Autodesk Fusion 360 part; units mm, degrees
(part 6 of 25)
  arc A2244 (43.1915, 31.5347) -> (43.1519, 31.5843) centre (43.1717, 31.5595) ccw
  arc A2245 (10.8585, 39.8209) -> (11.1125, 39.4716) centre (11.2256, 39.8209) ccw
  arc A2246 (43.2035, 31.5595) -> (43.14, 31.5595) centre (43.1717, 31.5595) ccw
  line L711 (42.8542, 31.3055) -> (43.1717, 31.5595)
  arc A2247 (42.037, 30.8928) -> (42.037, 30.9563) centre (42.037, 30.9246) ccw
  arc A2248 (42.037, 30.9563) -> (42.037, 30.8928) centre (42.037, 30.9246) ccw
  arc A2249 (23.3362, 25.2095) -> (23.2728, 25.2095) centre (23.3045, 25.2095) ccw
  arc A2250 (41.7195, 31.5912) -> (41.7195, 31.5278) centre (41.7195, 31.5595) ccw
  arc A2251 (42.8542, 30.4483) -> (42.8542, 30.3848) centre (42.8542, 30.4166) ccw
  arc A2252 (23.8454, 26.1303) -> (23.8454, 26.0668) centre (23.8454, 26.0985) ccw
  arc A2253 (24.2264, 26.1303) -> (24.2264, 26.0668) centre (24.2264, 26.0985) ccw
  arc A2254 (23.3362, 26.0985) -> (23.2728, 26.0985) centre (23.3045, 26.0985) ccw
  arc A2255 (42.037, 30.9245) -> (42.037, 31.5595) centre (42.037, 31.242) ccw
  arc A2256 (42.037, 31.5912) -> (42.037, 31.5278) centre (42.037, 31.5595) ccw
  line L712 (43.9972, 31.3055) -> (44.3147, 31.5595)
  line L713 (23.8454, 24.9555) -> (24.1629, 24.9555)
  arc A2257 (24.1629, 24.9238) -> (24.1629, 24.9872) centre (24.1629, 24.9555) ccw
  line L714 (23.3045, 26.0985) -> (23.3045, 25.2095)
  line L715 (43.1717, 31.5595) -> (43.1717, 30.4165)
  line L716 (42.8542, 30.4165) -> (43.4892, 30.4165)
  arc A2258 (42.8344, 31.3303) -> (42.874, 31.2807) centre (42.8542, 31.3055) ccw
  arc A2259 (42.3261, 30.4023) -> (42.3829, 30.4307) centre (42.3545, 30.4165) ccw
  arc A2260 (42.1289, 30.9387) -> (42.0721, 30.9103) centre (42.1005, 30.9245) ccw
  arc A2261 (23.0505, 24.9872) -> (23.0505, 24.9238) centre (23.0505, 24.9555) ccw
  arc A2262 (44.3465, 31.5595) -> (44.283, 31.5595) centre (44.3147, 31.5595) ccw
  arc A2263 (24.1629, 24.9555) -> (24.1629, 25.5905) centre (24.1629, 25.273) ccw
  arc A2264 (44.3345, 31.5347) -> (44.2949, 31.5843) centre (44.3147, 31.5595) ccw
  arc A2265 (41.6878, 30.4165) -> (41.7513, 30.4165) centre (41.7196, 30.4165) ccw
  arc A2266 (24.2264, 25.6223) -> (24.2264, 25.5588) centre (24.2264, 25.5906) ccw
  arc A2267 (24.2264, 25.5905) -> (24.2264, 26.0985) centre (24.2264, 25.8445) ccw
  line L717 (41.7195, 31.5595) -> (42.037, 31.5595)
  arc A2268 (11.9809, 39.4474) -> (12.0221, 39.4958) centre (12.0015, 39.4716) ccw
  arc A2269 (43.14, 30.4165) -> (43.2035, 30.4165) centre (43.1717, 30.4165) ccw
  arc A2270 (71.2481, 44.0055) -> (71.3116, 44.0055) centre (71.2798, 44.0055) ccw
  arc A2271 (23.8454, 24.9872) -> (23.8454, 24.9238) centre (23.8454, 24.9555) ccw
  arc A2272 (71.4704, 44.2278) -> (71.4704, 44.2913) centre (71.4704, 44.2596) ccw
  arc A2273 (44.283, 30.4165) -> (44.3465, 30.4165) centre (44.3147, 30.4165) ccw
  line L718 (24.2264, 25.5905) -> (23.9724, 25.5905)
  arc A2274 (23.2728, 25.2095) -> (23.3362, 25.2095) centre (23.3045, 25.2095) ccw
  arc A2275 (70.0405, 44.0373) -> (70.0405, 43.9738) centre (70.0405, 44.0055) ccw
  arc A2276 (56.1034, 43.8468) -> (56.1034, 43.9103) centre (56.1034, 43.8786) ccw
  arc A2277 (55.5636, 43.053) -> (55.6271, 43.053) centre (55.5954, 43.053) ccw
  arc A2278 (56.2621, 43.1165) -> (56.1986, 43.1165) centre (56.2304, 43.1165) ccw
  arc A2279 (56.2304, 43.1165) -> (55.9764, 43.3705) centre (55.9764, 43.1165) ccw
  arc A2280 (55.6271, 43.053) -> (55.5636, 43.053) centre (55.5954, 43.053) ccw
  arc A2281 (70.0405, 43.9738) -> (70.0405, 44.0373) centre (70.0405, 44.0055) ccw
  line L719 (55.0545, 43.8785) -> (55.0545, 42.9895)
  arc A2282 (71.2164, 31.3055) -> (71.4704, 31.5595) centre (71.2164, 31.5595) ccw
  arc A2283 (55.9764, 43.3387) -> (55.9764, 43.4023) centre (55.9764, 43.3705) ccw
  arc A2284 (70.0405, 44.0055) -> (70.2945, 44.2595) centre (70.0405, 44.2595) ccw
  arc A2285 (70.8048, 44.2682) -> (70.8659, 44.2508) centre (70.8354, 44.2595) ccw
  line L720 (70.8354, 31.9405) -> (70.8354, 32.4485)
  line L721 (70.8354, 44.2595) -> (71.4704, 44.2595)
  arc A2286 (70.3263, 32.4485) -> (70.2627, 32.4485) centre (70.2945, 32.4485) ccw
  line L722 (70.8354, 31.3055) -> (71.2164, 31.3055)
  line L723 (70.8354, 32.4485) -> (71.4704, 32.4485)
  arc A2287 (71.2164, 31.9088) -> (71.2164, 31.9722) centre (71.2164, 31.9405) ccw
  arc A2288 (70.3263, 31.5595) -> (70.2627, 31.5595) centre (70.2945, 31.5595) ccw
  arc A2289 (71.4704, 31.6865) -> (71.2164, 31.9405) centre (71.2164, 31.6865) ccw
  arc A2290 (71.4704, 32.4168) -> (71.4704, 32.4803) centre (71.4704, 32.4486) ccw
  line L724 (70.0405, 31.3055) -> (69.9135, 31.3055)
  arc A2291 (70.8036, 31.9405) -> (70.8671, 31.9405) centre (70.8354, 31.9405) ccw
  arc A2292 (70.8354, 44.2913) -> (70.8354, 44.2278) centre (70.8354, 44.2596) ccw
  arc A2293 (70.0405, 31.2738) -> (70.0405, 31.3373) centre (70.0405, 31.3056) ccw
  arc A2294 (71.4386, 31.6865) -> (71.5021, 31.6865) centre (71.4703, 31.6865) ccw
  arc A2295 (55.5954, 43.053) -> (56.2304, 43.053) centre (55.9129, 43.053) ccw
  line L725 (30.2566, 39.8145) -> (30.2566, 38.9255)
  line L726 (55.5954, 43.053) -> (55.5954, 43.3705)
  arc A2296 (56.1986, 43.053) -> (56.2621, 43.053) centre (56.2304, 43.053) ccw
  arc A2297 (55.0228, 42.9895) -> (55.0863, 42.9895) centre (55.0546, 42.9895) ccw
  arc A2298 (56.2621, 43.053) -> (56.1986, 43.053) centre (56.2304, 43.053) ccw
  arc A2299 (55.5954, 43.4023) -> (55.5954, 43.3387) centre (55.5954, 43.3705) ccw
  arc A2300 (71.3116, 44.5135) -> (71.2481, 44.5135) centre (71.2798, 44.5135) ccw
  arc A2301 (55.5636, 43.3705) -> (55.6271, 43.3705) centre (55.5954, 43.3705) ccw
  arc A2302 (54.8005, 42.7673) -> (54.8005, 42.7037) centre (54.8005, 42.7355) ccw
  arc A2303 (70.2627, 44.2595) -> (70.3263, 44.2595) centre (70.2945, 44.2595) ccw
  arc A2304 (71.2164, 31.2738) -> (71.2164, 31.3373) centre (71.2164, 31.3056) ccw
  arc A2305 (70.8671, 32.4485) -> (70.8036, 32.4485) centre (70.8354, 32.4485) ccw
  arc A2306 (71.4386, 31.5595) -> (71.5021, 31.5595) centre (71.4703, 31.5595) ccw
  arc A2307 (70.0405, 31.3373) -> (70.0405, 31.2738) centre (70.0405, 31.3056) ccw
  arc A2308 (71.2164, 31.3373) -> (71.2164, 31.2738) centre (71.2164, 31.3056) ccw
  arc A2309 (70.8354, 32.4803) -> (70.8354, 32.4168) centre (70.8354, 32.4486) ccw
  arc A2310 (55.0863, 42.9895) -> (55.0228, 42.9895) centre (55.0546, 42.9895) ccw
  arc A2311 (69.9135, 44.0373) -> (69.9135, 43.9738) centre (69.9135, 44.0055) ccw
  line L727 (55.5954, 43.3705) -> (55.9764, 43.3705)
  arc A2312 (71.5021, 31.5595) -> (71.4386, 31.5595) centre (71.4703, 31.5595) ccw
  arc A2313 (55.6271, 43.3705) -> (55.5636, 43.3705) centre (55.5954, 43.3705) ccw
  arc A2314 (71.2164, 31.9722) -> (71.2164, 31.9088) centre (71.2164, 31.9405) ccw
  arc A2315 (69.9135, 31.3373) -> (69.9135, 31.2738) centre (69.9135, 31.3056) ccw
  line L728 (70.0405, 44.0055) -> (69.9135, 44.0055)
  line L729 (71.2164, 31.9405) -> (70.8354, 31.9405)
  arc A2316 (70.8354, 31.3373) -> (70.8354, 31.2738) centre (70.8354, 31.3056) ccw
  arc A2317 (54.8005, 42.7037) -> (54.8005, 42.7673) centre (54.8005, 42.7355) ccw
  arc A2318 (71.5021, 31.6865) -> (71.4386, 31.6865) centre (71.4703, 31.6865) ccw
  arc A2319 (56.1986, 43.1165) -> (56.2621, 43.1165) centre (56.2304, 43.1165) ccw
  arc A2320 (70.2627, 31.5595) -> (70.3263, 31.5595) centre (70.2945, 31.5595) ccw
  arc A2321 (55.0863, 43.8785) -> (55.0228, 43.8785) centre (55.0546, 43.8785) ccw
  arc A2322 (54.8005, 42.7355) -> (55.0545, 42.9895) centre (54.8005, 42.9895) ccw
  line L730 (71.4704, 31.5595) -> (71.4704, 31.6865)
  arc A2323 (70.8354, 31.9722) -> (70.8354, 31.9088) centre (70.8354, 31.9405) ccw
  arc A2324 (70.0405, 31.3055) -> (70.2945, 31.5595) centre (70.0405, 31.5595) ccw
  arc A2325 (55.9764, 43.4023) -> (55.9764, 43.3387) centre (55.9764, 43.3705) ccw
  arc A2326 (58.1354, 31.623) -> (58.7704, 31.623) centre (58.4529, 31.623) ccw
  line L731 (30.7975, 39.8145) -> (31.4325, 39.8145)
  arc A2327 (54.6735, 42.7673) -> (54.6735, 42.7037) centre (54.6735, 42.7355) ccw
  arc A2328 (30.2884, 39.8145) -> (30.2249, 39.8145) centre (30.2567, 39.8145) ccw
  arc A2329 (30.7658, 39.6875) -> (30.8293, 39.6875) centre (30.7976, 39.6875) ccw
  arc A2330 (57.3405, 31.3055) -> (57.5945, 31.5595) centre (57.3405, 31.5595) ccw
  arc A2331 (30.7975, 39.8463) -> (30.7975, 39.7828) centre (30.7975, 39.8145) ccw
  arc A2332 (57.3405, 31.3373) -> (57.3405, 31.2738) centre (57.3405, 31.3056) ccw
  arc A2333 (57.3405, 31.2738) -> (57.3405, 31.3373) centre (57.3405, 31.3056) ccw
  arc A2334 (58.7704, 31.623) -> (58.1354, 31.623) centre (58.4529, 31.623) ccw
  arc A2335 (31.0844, 38.68) -> (31.1456, 38.663) centre (31.115, 38.6715) ccw
  arc A2336 (31.4325, 39.7828) -> (31.4325, 39.8463) centre (31.4325, 39.8145) ccw
  line L732 (7.8105, 49.0855) -> (7.6835, 49.0855)
  arc A2337 (7.8105, 49.0855) -> (8.0645, 49.3395) centre (7.8105, 49.3395) ccw
  arc A2338 (58.7386, 31.623) -> (58.8021, 31.623) centre (58.7704, 31.623) ccw
  arc A2339 (58.8021, 31.623) -> (58.7386, 31.623) centre (58.7704, 31.623) ccw
  arc A2340 (57.6263, 32.4485) -> (57.5628, 32.4485) centre (57.5945, 32.4485) ccw
  arc A2341 (58.1036, 31.623) -> (58.1671, 31.623) centre (58.1354, 31.623) ccw
  arc A2342 (58.7386, 32.1945) -> (58.6751, 32.1945) centre (58.7069, 32.1945) ccw
  line L733 (31.4325, 39.8145) -> (31.115, 38.6715)
  arc A2343 (7.8105, 49.0538) -> (7.8105, 49.1173) centre (7.8105, 49.0856) ccw
  arc A2344 (9.2404, 49.5618) -> (9.2404, 49.6253) centre (9.2404, 49.5936) ccw
  arc A2345 (30.0026, 38.6715) -> (30.2566, 38.9255) centre (30.0026, 38.9255) ccw
  arc A2346 (29.8756, 38.7033) -> (29.8756, 38.6397) centre (29.8756, 38.6715) ccw
  arc A2347 (30.2249, 38.9255) -> (30.2884, 38.9255) centre (30.2567, 38.9255) ccw
  arc A2348 (7.8105, 49.1173) -> (7.8105, 49.0538) centre (7.8105, 49.0856) ccw
  arc A2349 (8.6371, 49.911) -> (8.5736, 49.911) centre (8.6054, 49.911) ccw
  arc A2350 (8.0963, 49.3395) -> (8.0328, 49.3395) centre (8.0646, 49.3395) ccw
  arc A2351 (58.6751, 32.1945) -> (58.7386, 32.1945) centre (58.7069, 32.1945) ccw
  line L734 (56.2304, 43.1165) -> (56.2304, 43.053)
  line L735 (9.2404, 49.5935) -> (8.8594, 49.5935)
  arc A2352 (58.1989, 32.1945) -> (58.7069, 32.1945) centre (58.4529, 32.1945) ccw
  line L736 (57.5945, 32.4485) -> (57.5945, 31.5595)
  arc A2353 (8.8594, 49.6253) -> (8.8594, 49.5618) centre (8.8594, 49.5936) ccw
  line L737 (8.0645, 50.2285) -> (8.0645, 49.3395)
  line L738 (30.7975, 39.6875) -> (30.7975, 39.8145)
  arc A2354 (8.6054, 49.8475) -> (8.8594, 49.5935) centre (8.8594, 49.8475) ccw
  arc A2355 (30.8293, 39.8145) -> (30.7658, 39.8145) centre (30.7976, 39.8145) ccw
  arc A2356 (57.2135, 31.3373) -> (57.2135, 31.2738) centre (57.2135, 31.3056) ccw
  arc A2357 (30.0026, 38.7033) -> (30.0026, 38.6397) centre (30.0026, 38.6715) ccw
  arc A2358 (30.2884, 38.9255) -> (30.2249, 38.9255) centre (30.2567, 38.9255) ccw
  arc A2359 (58.2306, 32.1945) -> (58.1671, 32.1945) centre (58.1989, 32.1945) ccw
  arc A2360 (58.1671, 31.623) -> (58.1036, 31.623) centre (58.1354, 31.623) ccw
  line L739 (54.8005, 42.7355) -> (54.6735, 42.7355)
  arc A2361 (8.0328, 49.3395) -> (8.0963, 49.3395) centre (8.0646, 49.3395) ccw
  arc A2362 (56.1034, 43.8785) -> (55.5954, 43.3705) centre (56.1034, 43.3705) ccw
  arc A2363 (57.6263, 31.5595) -> (57.5628, 31.5595) centre (57.5945, 31.5595) ccw
  arc A2364 (31.4631, 39.806) -> (31.4019, 39.823) centre (31.4325, 39.8145) ccw
  line L740 (30.0026, 38.6715) -> (29.8756, 38.6715)
  arc A2365 (7.6835, 49.1173) -> (7.6835, 49.0538) centre (7.6835, 49.0856) ccw
  arc A2366 (8.6371, 49.8475) -> (8.5736, 49.8475) centre (8.6054, 49.8475) ccw
  arc A2367 (8.8594, 49.5618) -> (8.8594, 49.6253) centre (8.8594, 49.5936) ccw
  arc A2368 (58.1671, 32.1945) -> (58.2306, 32.1945) centre (58.1989, 32.1945) ccw
  arc A2369 (57.5628, 31.5595) -> (57.6263, 31.5595) centre (57.5945, 31.5595) ccw
  line L741 (8.6054, 49.8475) -> (8.6054, 49.911)
  arc A2370 (8.0963, 50.2285) -> (8.0328, 50.2285) centre (8.0646, 50.2285) ccw
  line L742 (57.3405, 31.3055) -> (57.2135, 31.3055)
  arc A2371 (30.0026, 38.6397) -> (30.0026, 38.7033) centre (30.0026, 38.6715) ccw
  arc A2372 (58.7069, 32.1945) -> (58.1989, 32.1945) centre (58.4529, 32.1945) ccw
  arc A2373 (45.3073, 23.3045) -> (45.2437, 23.3045) centre (45.2755, 23.3045) ccw
  arc A2374 (31.8167, 35.0342) -> (31.8738, 35.0063) centre (31.8453, 35.0203) ccw
  arc A2375 (31.9722, 35.433) -> (31.9088, 35.433) centre (31.9405, 35.433) ccw
  arc A2376 (31.4308, 35.0305) -> (31.3707, 35.01) centre (31.4008, 35.0203) ccw
  line L743 (30.1625, 34.8615) -> (30.7975, 34.8615)
  arc A2377 (9.2721, 49.911) -> (9.2086, 49.911) centre (9.2404, 49.911) ccw
  arc A2378 (31.623, 35.9727) -> (31.623, 36.0363) centre (31.623, 36.0045) ccw
  arc A2379 (29.6534, 36.0045) -> (29.5899, 36.0045) centre (29.6217, 36.0045) ccw
  arc A2380 (31.3442, 35.1353) -> (31.3938, 35.0957) centre (31.369, 35.1155) ccw
  arc A2381 (9.2721, 49.5935) -> (9.2086, 49.5935) centre (9.2404, 49.5935) ccw
  arc A2382 (8.7324, 49.0855) -> (9.2404, 49.5935) centre (8.7324, 49.5935) ccw
  arc A2383 (29.6534, 35.1155) -> (29.5899, 35.1155) centre (29.6217, 35.1155) ccw
  arc A2384 (30.4998, 35.9797) -> (30.4602, 36.0293) centre (30.48, 36.0045) ccw
  arc A2385 (31.8738, 35.8597) -> (31.8167, 35.8318) centre (31.8453, 35.8457) ccw
  arc A2386 (31.9088, 35.433) -> (31.9722, 35.433) centre (31.9405, 35.433) ccw
  line L744 (29.6216, 36.0045) -> (29.6216, 35.1155)
  arc A2387 (29.5899, 35.1155) -> (29.6534, 35.1155) centre (29.6217, 35.1155) ccw
  arc A2388 (31.4008, 35.8458) -> (31.3055, 35.433) centre (32.2475, 35.4329) ccw
  line L745 (30.1625, 35.7505) -> (30.48, 36.0045)
  line L746 (45.0215, 22.1615) -> (44.8945, 22.1615)
  arc A2389 (31.623, 34.8615) -> (31.8453, 35.0203) centre (31.623, 35.0965) ccw
  arc A2390 (31.623, 36.0363) -> (31.623, 35.9727) centre (31.623, 36.0045) ccw
  arc A2391 (29.3676, 34.8297) -> (29.3676, 34.8933) centre (29.3676, 34.8615) ccw
  arc A2392 (30.1427, 35.7753) -> (30.1823, 35.7257) centre (30.1625, 35.7505) ccw
  arc A2393 (30.7975, 34.8297) -> (30.7975, 34.8933) centre (30.7975, 34.8615) ccw
  arc A2394 (31.3373, 35.433) -> (31.2738, 35.433) centre (31.3056, 35.433) ccw
  arc A2395 (31.3722, 35.0063) -> (31.4293, 35.0342) centre (31.4008, 35.0203) ccw
  arc A2396 (45.0215, 22.1615) -> (45.2755, 22.4155) centre (45.0215, 22.4155) ccw
  arc A2397 (44.8945, 22.1932) -> (44.8945, 22.1298) centre (44.8945, 22.1615) ccw
  arc A2398 (45.3073, 22.4155) -> (45.2437, 22.4155) centre (45.2755, 22.4155) ccw
  arc A2399 (31.8753, 35.01) -> (31.8152, 35.0305) centre (31.8453, 35.0203) ccw
  arc A2400 (31.8453, 35.0203) -> (31.9405, 35.433) centre (30.9988, 35.4329) ccw
  arc A2401 (31.623, 36.0045) -> (31.4008, 35.8458) centre (31.623, 35.7696) ccw
  arc A2402 (31.3055, 35.433) -> (31.4008, 35.0203) centre (32.2472, 35.4331) ccw
  arc A2403 (30.4483, 34.8615) -> (30.5117, 34.8615) centre (30.48, 34.8615) ccw
  arc A2404 (31.8152, 35.8355) -> (31.8753, 35.856) centre (31.8453, 35.8458) ccw
  line L747 (45.2755, 23.3045) -> (45.2755, 22.4155)
  arc A2405 (9.2086, 49.911) -> (9.2721, 49.911) centre (9.2404, 49.911) ccw
  arc A2406 (29.3676, 34.8615) -> (29.6216, 35.1155) centre (29.3676, 35.1155) ccw
  arc A2407 (9.2086, 49.5935) -> (9.2721, 49.5935) centre (9.2404, 49.5935) ccw
  arc A2408 (45.2437, 22.4155) -> (45.3073, 22.4155) centre (45.2755, 22.4155) ccw
  line L748 (31.369, 35.1155) -> (31.877, 35.7505)
  arc A2409 (31.4008, 35.0203) -> (31.623, 34.8615) centre (31.623, 35.0964) ccw
  arc A2410 (31.3707, 35.856) -> (31.4308, 35.8355) centre (31.4007, 35.8458) ccw
  arc A2411 (29.2406, 34.8933) -> (29.2406, 34.8297) centre (29.2406, 34.8615) ccw
  arc A2412 (31.623, 34.8933) -> (31.623, 34.8297) centre (31.623, 34.8615) ccw
  arc A2413 (8.5736, 49.8475) -> (8.6371, 49.8475) centre (8.6054, 49.8475) ccw
  arc A2414 (31.2738, 35.433) -> (31.3373, 35.433) centre (31.3056, 35.433) ccw
  arc A2415 (31.623, 34.8297) -> (31.623, 34.8933) centre (31.623, 34.8615) ccw
  arc A2416 (30.1625, 34.8933) -> (30.1625, 34.8297) centre (30.1625, 34.8615) ccw
  line L749 (30.48, 36.0045) -> (30.48, 34.8615)
  arc A2417 (9.2404, 49.911) -> (8.6054, 49.911) centre (8.9229, 49.911) ccw
  arc A2418 (29.3676, 34.8933) -> (29.3676, 34.8297) centre (29.3676, 34.8615) ccw
  arc A2419 (45.0215, 22.1932) -> (45.0215, 22.1298) centre (45.0215, 22.1615) ccw
  arc A2420 (31.4293, 35.8318) -> (31.3722, 35.8597) centre (31.4007, 35.8457) ccw
  arc A2421 (30.5117, 36.0045) -> (30.4483, 36.0045) centre (30.48, 36.0045) ccw
  arc A2422 (8.7324, 49.1173) -> (8.7324, 49.0538) centre (8.7324, 49.0856) ccw
  line L750 (9.2404, 49.911) -> (9.2404, 49.5935)
  line L751 (29.3676, 34.8615) -> (29.2406, 34.8615)
  arc A2423 (8.5736, 49.911) -> (8.6371, 49.911) centre (8.6054, 49.911) ccw
  arc A2424 (31.9405, 35.433) -> (31.8453, 35.8458) centre (30.9986, 35.4332) ccw
  line L752 (46.9594, 22.1615) -> (47.5944, 22.1615)
  arc A2425 (46.1537, 23.2797) -> (46.114, 23.3293) centre (46.1339, 23.3045) ccw
  arc A2426 (18.0199, 16.8275) -> (18.0199, 16.7005) centre (18.0199, 16.764) ccw
  arc A2427 (19.9488, 16.8051) -> (20.0456, 16.7229) centre (19.9972, 16.764) ccw
  arc A2428 (18.1822, 16.9898) -> (18.3092, 16.9898) centre (18.2457, 16.9898) ccw
  line L753 (20.477, 17.3284) -> (19.9972, 16.764)
  arc A2429 (19.1999, 17.78) -> (19.0729, 17.78) centre (19.1364, 17.78) ccw
  arc A2430 (31.8453, 35.8458) -> (31.623, 36.0045) centre (31.6231, 35.7696) ccw
  arc A2431 (20.5253, 17.2873) -> (20.4286, 17.3696) centre (20.477, 17.3284) ccw
  arc A2432 (47.2451, 22.1615) -> (47.3086, 22.1615) centre (47.2769, 22.1615) ccw
  arc A2433 (18.3092, 17.78) -> (18.1822, 17.78) centre (18.2457, 17.78) ccw
  line L754 (11.1718, 33.7058) -> (11.8209, 33.7058)
  arc A2434 (46.1021, 22.1615) -> (46.1656, 22.1615) centre (46.1339, 22.1615) ccw
  arc A2435 (20.3076, 17.78) -> (19.9972, 17.5542) centre (20.3076, 17.4537) ccw
  arc A2436 (19.9368, 17.5738) -> (20.0576, 17.5347) centre (19.9972, 17.5542) ccw
  line L755 (45.8164, 22.1615) -> (46.4514, 22.1615)
  arc A2437 (20.6251, 17.526) -> (20.4981, 17.526) centre (20.5616, 17.526) ccw
  arc A2438 (20.5616, 16.7005) -> (20.5616, 16.8275) centre (20.5616, 16.764) ccw
  arc A2439 (10.1092, 34.8742) -> (10.0584, 34.8742) centre (10.0838, 34.8742) ccw
  arc A2440 (18.8145, 17.6038) -> (18.8939, 17.5046) centre (18.8542, 17.5542) ccw
  arc A2441 (19.0729, 16.764) -> (19.1999, 16.764) centre (19.1364, 16.764) ccw
  arc A2442 (20.477, 17.3284) -> (20.5616, 17.526) centre (20.2888, 17.5259) ccw
  arc A2443 (18.3092, 16.9898) -> (18.1822, 16.9898) centre (18.2457, 16.9898) ccw
  arc A2444 (45.7965, 23.0753) -> (45.8362, 23.0257) centre (45.8163, 23.0505) ccw
  arc A2445 (17.907, 16.8275) -> (17.907, 16.7005) centre (17.907, 16.764) ccw
  arc A2446 (19.9972, 16.8275) -> (19.9972, 16.7005) centre (19.9972, 16.764) ccw
  arc A2447 (19.4186, 16.7005) -> (19.4186, 16.8275) centre (19.4186, 16.764) ccw
  line L756 (18.0199, 16.764) -> (17.907, 16.764)
  arc A2448 (19.1761, 17.7304) -> (19.0967, 17.8296) centre (19.1364, 17.78) ccw
  arc A2449 (11.4709, 33.7058) -> (11.5217, 33.7058) centre (11.4963, 33.7058) ccw
  line L757 (10.7329, 33.7058) -> (10.3434, 34.4198)
  arc A2450 (10.0584, 33.7058) -> (10.1092, 33.7058) centre (10.0838, 33.7058) ccw
  line L758 (18.8542, 17.5542) -> (19.1364, 17.78)
  line L759 (10.0838, 33.7058) -> (10.0838, 34.8742)
  arc A2451 (20.4332, 17.3744) -> (20.5208, 17.2825) centre (20.477, 17.3285) ccw
  arc A2452 (18.8542, 16.8275) -> (18.8542, 16.7005) centre (18.8542, 16.764) ccw
  line L760 (45.8164, 23.0505) -> (46.1339, 23.3045)
  arc A2453 (46.9594, 22.1932) -> (46.9594, 22.1298) centre (46.9594, 22.1615) ccw
  line L761 (19.1364, 17.78) -> (19.1364, 16.764)
  arc A2454 (20.5616, 17.526) -> (20.3076, 17.78) centre (20.3076, 17.526) ccw
  arc A2455 (18.0199, 16.7005) -> (18.0199, 16.8275) centre (18.0199, 16.764) ccw
  arc A2456 (11.1559, 34.6344) -> (11.1876, 34.5947) centre (11.1717, 34.6146) ccw
  arc A2457 (46.4514, 22.1298) -> (46.4514, 22.1932) centre (46.4514, 22.1615) ccw
  arc A2458 (18.0199, 16.764) -> (18.2457, 16.9898) centre (18.0199, 16.9898) ccw
  line L762 (19.9972, 16.764) -> (20.5616, 16.764)
  arc A2459 (31.9018, 35.7307) -> (31.8522, 35.7703) centre (31.877, 35.7505) ccw
  arc A2460 (47.3086, 23.3045) -> (47.2451, 23.3045) centre (47.2769, 23.3045) ccw
  line L763 (47.2769, 23.3045) -> (47.2769, 22.1615)
  arc A2461 (45.8164, 22.1932) -> (45.8164, 22.1298) centre (45.8164, 22.1615) ccw
  arc A2462 (47.5944, 22.1298) -> (47.5944, 22.1932) centre (47.5944, 22.1615) ccw
  line L764 (18.2457, 17.78) -> (18.2457, 16.9898)
  arc A2463 (46.9395, 23.0753) -> (46.9792, 23.0257) centre (46.9594, 23.0505) ccw
  arc A2464 (20.4981, 17.526) -> (20.6251, 17.526) centre (20.5616, 17.526) ccw
  arc A2465 (46.1656, 23.3045) -> (46.1021, 23.3045) centre (46.1339, 23.3045) ccw
  line L765 (18.8542, 16.764) -> (19.4186, 16.764)
  arc A2466 (47.2967, 23.2797) -> (47.257, 23.3293) centre (47.2769, 23.3045) ccw
  arc A2467 (45.0215, 22.1298) -> (45.0215, 22.1932) centre (45.0215, 22.1615) ccw
  line L766 (46.1339, 23.3045) -> (46.1339, 22.1615)
  line L767 (46.9594, 23.0505) -> (47.2769, 23.3045)
  arc A2468 (20.3076, 17.7165) -> (20.3076, 17.8435) centre (20.3076, 17.78) ccw
  arc A2469 (20.3076, 17.8435) -> (20.3076, 17.7165) centre (20.3076, 17.78) ccw
  arc A2470 (11.5122, 34.8544) -> (11.4804, 34.894) centre (11.4963, 34.8742) ccw
  arc A2471 (11.1718, 33.7312) -> (11.1718, 33.6804) centre (11.1718, 33.7058) ccw
  arc A2472 (11.8209, 33.6804) -> (11.8209, 33.7312) centre (11.8209, 33.7058) ccw
  line L768 (4.4958, 8.0518) -> (3.9878, 8.0518)
  arc A2473 (12.3825, 8.0328) -> (12.3825, 8.0963) centre (12.3825, 8.0646) ccw
  arc A2474 (4.4958, 8.02) -> (4.4958, 8.0836) centre (4.4958, 8.0518) ccw
  arc A2475 (3.5052, 8.02) -> (3.5052, 8.0836) centre (3.5052, 8.0518) ccw
  line L769 (4.9759, 9.1948) -> (5.2934, 9.1948)
  arc A2476 (5.5791, 8.8773) -> (5.6426, 8.8773) centre (5.6108, 8.8773) ccw
  arc A2477 (3.029, 9.1948) -> (2.9655, 9.1948) centre (2.9973, 9.1948) ccw
  arc A2478 (2.9972, 8.0836) -> (2.9972, 8.02) centre (2.9972, 8.0518) ccw
  line L770 (10.7329, 34.8742) -> (10.0838, 34.1602)
  arc A2479 (10.7517, 34.8571) -> (10.7141, 34.8913) centre (10.7329, 34.8742) ccw
  arc A2480 (6.4427, 8.0518) -> (6.5062, 8.0518) centre (6.4745, 8.0518) ccw
  arc A2481 (5.2934, 9.1631) -> (5.2934, 9.2266) centre (5.2934, 9.1949) ccw
  line L771 (5.2934, 8.0518) -> (4.9759, 8.0518)
  line L772 (3.9878, 8.0518) -> (3.9878, 9.1948)
  arc A2482 (5.2934, 8.0518) -> (5.6109, 8.3693) centre (5.2934, 8.3693) ccw
  arc A2483 (6.1371, 8.9656) -> (6.1768, 8.916) centre (6.157, 8.9408) ccw
  line L773 (6.157, 8.9408) -> (6.4745, 9.1948)
  arc A2484 (6.792, 8.02) -> (6.792, 8.0836) centre (6.792, 8.0518) ccw
  arc A2485 (5.6426, 8.3693) -> (5.5791, 8.3693) centre (5.6108, 8.3693) ccw
  line L774 (6.4745, 9.1948) -> (6.4745, 8.0518)
  line L775 (5.6109, 8.8773) -> (5.6109, 8.3693)
  arc A2486 (5.2934, 8.0836) -> (5.2934, 8.02) centre (5.2934, 8.0518) ccw
  arc A2487 (10.065, 34.1773) -> (10.1026, 34.1431) centre (10.0838, 34.1602) ccw
  arc A2488 (2.9655, 8.0518) -> (3.029, 8.0518) centre (2.9973, 8.0518) ccw
  arc A2489 (5.5791, 8.3693) -> (5.6426, 8.3693) centre (5.6108, 8.3693) ccw
  line L776 (3.9878, 8.6868) -> (4.3688, 8.6868)
  arc A2490 (5.6426, 8.8773) -> (5.5791, 8.8773) centre (5.6108, 8.8773) ccw
  arc A2491 (10.7106, 33.6936) -> (10.7552, 33.718) centre (10.7329, 33.7058) ccw
  line L777 (11.1718, 34.6146) -> (11.4963, 34.8742)
  line L778 (6.157, 8.0518) -> (6.792, 8.0518)
  arc A2492 (15.6693, 8.0328) -> (15.6693, 8.0963) centre (15.6693, 8.0646) ccw
  arc A2493 (3.956, 8.0518) -> (4.0195, 8.0518) centre (3.9878, 8.0518) ccw
  line L779 (11.8745, 9.2075) -> (11.8745, 8.0645)
  arc A2494 (5.2934, 9.2266) -> (5.2934, 9.1631) centre (5.2934, 9.1949) ccw
  arc A2495 (6.157, 8.0836) -> (6.157, 8.02) centre (6.157, 8.0518) ccw
  arc A2496 (3.9878, 8.0836) -> (3.9878, 8.02) centre (3.9878, 8.0518) ccw
  line L780 (2.9972, 8.0518) -> (3.5052, 8.0518)
  line L781 (3.9878, 9.1948) -> (4.4958, 9.1948)
  arc A2497 (4.4958, 9.1631) -> (4.4958, 9.2266) centre (4.4958, 9.1949) ccw
  arc A2498 (5.2934, 8.02) -> (5.2934, 8.0836) centre (5.2934, 8.0518) ccw
  arc A2499 (4.0195, 9.1948) -> (3.956, 9.1948) centre (3.9878, 9.1948) ccw
  arc A2500 (3.9878, 9.2266) -> (3.9878, 9.1631) centre (3.9878, 9.1949) ccw
  line L782 (11.4963, 34.8742) -> (11.4963, 33.7058)
  arc A2501 (4.3688, 8.655) -> (4.3688, 8.7186) centre (4.3688, 8.6868) ccw
  line L783 (4.9759, 8.0518) -> (4.9759, 9.1948)
  arc A2502 (11.5217, 34.8742) -> (11.4709, 34.8742) centre (11.4963, 34.8742) ccw
  arc A2503 (4.9759, 9.2266) -> (4.9759, 9.1631) centre (4.9759, 9.1949) ccw
  arc A2504 (4.9759, 8.0836) -> (4.9759, 8.02) centre (4.9759, 8.0518) ccw
  arc A2505 (3.9878, 8.7186) -> (3.9878, 8.655) centre (3.9878, 8.6868) ccw
  arc A2506 (6.4943, 9.17) -> (6.4546, 9.2196) centre (6.4745, 9.1948) ccw
  arc A2507 (10.3657, 34.432) -> (10.3211, 34.4077) centre (10.3434, 34.4199) ccw
  line L784 (13.3731, 8.0645) -> (12.8651, 8.0645)
  arc A2508 (5.6109, 8.8773) -> (5.2934, 9.1948) centre (5.2934, 8.8773) ccw
  arc A2509 (15.701, 8.9218) -> (15.6375, 8.9217) centre (15.6692, 8.9218) ccw
  arc A2510 (6.5062, 9.1948) -> (6.4427, 9.1948) centre (6.4745, 9.1948) ccw
  arc A2511 (5.0076, 9.1948) -> (4.9441, 9.1948) centre (4.9759, 9.1948) ccw
  arc A2512 (4.9441, 8.0518) -> (5.0076, 8.0518) centre (4.9759, 8.0518) ccw
  line L785 (2.9972, 9.1948) -> (2.9972, 8.0518)
  arc A2513 (12.8968, 9.2075) -> (12.8333, 9.2075) centre (12.8651, 9.2075) ccw
  arc A2514 (14.1707, 9.1757) -> (14.1707, 9.2393) centre (14.1707, 9.2075) ccw
  arc A2515 (14.4564, 8.89) -> (14.5199, 8.89) centre (14.4881, 8.89) ccw
  line L786 (76.708, 14.5415) -> (76.3905, 14.5415)
  arc A2516 (15.0101, 8.0851) -> (15.0584, 8.0439) centre (15.0343, 8.0645) ccw
  arc A2517 (76.3905, 14.5733) -> (76.3905, 14.5098) centre (76.3905, 14.5416) ccw
  arc A2518 (14.1707, 9.2393) -> (14.1707, 9.1757) centre (14.1707, 9.2075) ccw
  arc A2519 (13.8214, 8.0645) -> (13.8849, 8.0645) centre (13.8532, 8.0645) ccw
  arc A2520 (14.1707, 8.0963) -> (14.1707, 8.0328) centre (14.1707, 8.0646) ccw
  arc A2521 (12.8651, 9.2393) -> (12.8651, 9.1757) centre (12.8651, 9.2075) ccw
  arc A2522 (77.5054, 14.9473) -> (77.545, 14.8977) centre (77.5252, 14.9225) ccw
  line L787 (77.5252, 14.9225) -> (77.8427, 15.1765)
  arc A2523 (76.3588, 14.0335) -> (76.4223, 14.0335) centre (76.3906, 14.0335) ccw
  line L788 (15.574, 8.6995) -> (15.0343, 8.0645)
  arc A2524 (13.3731, 9.1757) -> (13.3731, 9.2393) centre (13.3731, 9.2075) ccw
  arc A2525 (14.4564, 8.382) -> (14.5199, 8.382) centre (14.4881, 8.382) ccw
  arc A2526 (13.8532, 8.0963) -> (13.8532, 8.0328) centre (13.8532, 8.0646) ccw
  arc A2527 (76.3905, 15.2083) -> (76.3905, 15.1448) centre (76.3905, 15.1766) ccw
  line L789 (76.3905, 15.1765) -> (76.708, 15.1765)
  arc A2528 (76.7999, 14.5557) -> (76.7431, 14.5273) centre (76.7715, 14.5415) ccw
  arc A2529 (76.708, 15.1448) -> (76.708, 15.2083) centre (76.708, 15.1766) ccw
  line L790 (13.8532, 9.2075) -> (14.1707, 9.2075)
  line L791 (14.4882, 8.89) -> (14.4882, 8.382)
  line L792 (12.8651, 9.2075) -> (13.3731, 9.2075)
  arc A2530 (15.5521, 8.7225) -> (15.5959, 8.6765) centre (15.574, 8.6995) ccw
  line L793 (11.8745, 8.0645) -> (12.3825, 8.0645)
  arc A2531 (15.3835, 9.2075) -> (15.0343, 8.9535) centre (15.3835, 8.8404) ccw
  arc A2532 (12.8651, 8.0963) -> (12.8651, 8.0328) centre (12.8651, 8.0646) ccw
  line L794 (12.8651, 8.0645) -> (12.8651, 9.2075)
  arc A2533 (14.1707, 8.0328) -> (14.1707, 8.0963) centre (14.1707, 8.0646) ccw
  arc A2534 (11.9063, 9.2075) -> (11.8428, 9.2075) centre (11.8746, 9.2075) ccw
  arc A2535 (76.708, 14.5098) -> (76.708, 14.5733) centre (76.708, 14.5416) ccw
  arc A2536 (14.5199, 8.89) -> (14.4564, 8.89) centre (14.4881, 8.89) ccw
  arc A2537 (11.8428, 8.0645) -> (11.9063, 8.0645) centre (11.8746, 8.0645) ccw
  arc A2538 (15.3835, 9.1757) -> (15.3835, 9.2393) centre (15.3835, 9.2075) ccw
  arc A2539 (12.8333, 8.0645) -> (12.8968, 8.0645) centre (12.8651, 8.0645) ccw
  arc A2540 (77.8745, 15.1765) -> (77.811, 15.1765) centre (77.8428, 15.1765) ccw
  arc A2541 (14.4882, 8.89) -> (14.1707, 9.2075) centre (14.1707, 8.89) ccw
  arc A2542 (15.6375, 8.9218) -> (15.701, 8.9218) centre (15.6693, 8.9218) ccw
  arc A2543 (13.8849, 9.2075) -> (13.8214, 9.2075) centre (13.8532, 9.2075) ccw
  arc A2544 (15.3835, 9.2393) -> (15.3835, 9.1757) centre (15.3835, 9.2075) ccw
  line L795 (14.1707, 8.0645) -> (13.8532, 8.0645)
  line L796 (77.5252, 14.0335) -> (78.1602, 14.0335)
  arc A2545 (14.1707, 8.0645) -> (14.4882, 8.382) centre (14.1707, 8.382) ccw
  arc A2546 (78.1602, 14.0017) -> (78.1602, 14.0653) centre (78.1602, 14.0335) ccw
  arc A2547 (15.574, 8.6995) -> (15.6693, 8.9218) centre (15.3624, 8.9218) ccw
  arc A2548 (11.8745, 8.0963) -> (11.8745, 8.0328) centre (11.8745, 8.0646) ccw
  arc A2549 (15.0343, 8.0963) -> (15.0343, 8.0328) centre (15.0343, 8.0646) ccw
  arc A2550 (15.6693, 8.9218) -> (15.3835, 9.2075) centre (15.3835, 8.9217) ccw
  line L797 (12.8651, 8.6995) -> (13.2461, 8.6995)
  arc A2551 (12.8651, 8.7313) -> (12.8651, 8.6677) centre (12.8651, 8.6995) ccw
  line L798 (13.8532, 8.0645) -> (13.8532, 9.2075)
  arc A2552 (15.5982, 8.6789) -> (15.5498, 8.7201) centre (15.574, 8.6995) ccw
  arc A2553 (13.3731, 8.0328) -> (13.3731, 8.0963) centre (13.3731, 8.0646) ccw
  arc A2554 (76.9971, 14.0193) -> (77.0539, 14.0477) centre (77.0255, 14.0335) ccw
  arc A2555 (13.8532, 9.2393) -> (13.8532, 9.1757) centre (13.8532, 9.2075) ccw
  arc A2556 (14.5199, 8.382) -> (14.4564, 8.382) centre (14.4881, 8.382) ccw
  line L799 (76.3905, 14.0335) -> (76.3905, 15.1765)
  arc A2557 (15.0041, 8.9633) -> (15.0645, 8.9437) centre (15.0343, 8.9535) ccw
  line L800 (15.0343, 8.0645) -> (15.6693, 8.0645)
  arc A2558 (76.708, 14.5415) -> (76.708, 15.1765) centre (76.708, 14.859) ccw
  arc A2559 (13.2461, 8.6677) -> (13.2461, 8.7313) centre (13.2461, 8.6995) ccw
  arc A2560 (10.8248, 9.6965) -> (10.5391, 9.9822) centre (10.5391, 9.6965) ccw
  arc A2561 (10.8566, 9.6965) -> (10.7931, 9.6964) centre (10.8249, 9.6965) ccw
  arc A2562 (76.4223, 15.1765) -> (76.3588, 15.1765) centre (76.3906, 15.1765) ccw
  arc A2563 (10.1596, 9.738) -> (10.22, 9.7184) centre (10.1898, 9.7282) ccw
  arc A2564 (10.7538, 9.4536) -> (10.7054, 9.4948) centre (10.7296, 9.4742) ccw
  arc A2565 (9.0869, 9.9822) -> (9.0234, 9.9822) centre (9.0552, 9.9822) ccw
  arc A2566 (10.7296, 9.4742) -> (10.8248, 9.6965) centre (10.5179, 9.6964) ccw
  arc A2567 (10.5391, 9.9505) -> (10.5391, 10.014) centre (10.5391, 9.9823) ccw
  arc A2568 (77.9062, 28.2892) -> (77.9062, 28.2258) centre (77.9062, 28.2575) ccw
  arc A2569 (10.5391, 9.9822) -> (10.1898, 9.7282) centre (10.5391, 9.6151) ccw
  arc A2570 (10.7077, 9.4972) -> (10.7515, 9.4512) centre (10.7296, 9.4742) ccw
  line L801 (77.0255, 14.0335) -> (76.7715, 14.5415)
  arc A2571 (77.5252, 14.0653) -> (77.5252, 14.0017) centre (77.5252, 14.0335) ccw
  arc A2572 (10.5391, 10.014) -> (10.5391, 9.9505) centre (10.5391, 9.9823) ccw
  arc A2573 (76.708, 28.2258) -> (76.708, 28.2892) centre (76.708, 28.2575) ccw
  arc A2574 (9.0551, 9.379) -> (9.0551, 9.3155) centre (9.0551, 9.3473) ccw
  line L802 (77.5252, 27.1145) -> (77.8427, 27.1145)
  arc A2575 (77.5252, 28.2892) -> (77.5252, 28.2258) centre (77.5252, 28.2575) ccw
  arc A2576 (77.8427, 27.1145) -> (77.8427, 27.7495) centre (77.8427, 27.432) ccw
  arc A2577 (76.708, 27.6543) -> (76.708, 27.5908) centre (76.708, 27.6226) ccw
  arc A2578 (76.708, 27.5908) -> (76.708, 27.6543) centre (76.708, 27.6226) ccw
  arc A2579 (77.8625, 15.1517) -> (77.8229, 15.2013) centre (77.8427, 15.1765) ccw
  line L803 (76.708, 27.6225) -> (76.3905, 27.6225)
  arc A2580 (10.1898, 8.871) -> (10.1898, 8.8074) centre (10.1898, 8.8392) ccw
  arc A2581 (9.0551, 10.014) -> (9.0551, 9.9505) centre (9.0551, 9.9823) ccw
  arc A2582 (9.0234, 8.8392) -> (9.0869, 8.8392) centre (9.0552, 8.8392) ccw
  line L804 (77.9062, 27.7495) -> (77.6522, 27.7495)
  arc A2583 (77.9062, 28.2258) -> (77.9062, 28.2892) centre (77.9062, 28.2575) ccw
  arc A2584 (76.9971, 27.1003) -> (77.0539, 27.1287) centre (77.0255, 27.1145) ccw
  line L805 (9.3726, 9.3472) -> (9.0551, 9.3472)
  arc A2585 (77.811, 14.0335) -> (77.8745, 14.0335) centre (77.8428, 14.0335) ccw
  arc A2586 (9.3726, 9.379) -> (9.3726, 9.3155) centre (9.3726, 9.3473) ccw
  line L806 (76.3905, 27.1145) -> (76.3905, 28.2575)
  arc A2587 (9.3726, 9.3155) -> (9.3726, 9.379) centre (9.3726, 9.3473) ccw
  arc A2588 (76.7999, 27.6367) -> (76.7431, 27.6083) centre (76.7715, 27.6225) ccw
  arc A2589 (77.8427, 27.0828) -> (77.8427, 27.1462) centre (77.8427, 27.1145) ccw
  arc A2590 (77.8427, 27.1462) -> (77.8427, 27.0828) centre (77.8427, 27.1145) ccw
  arc A2591 (9.6617, 8.825) -> (9.7185, 8.8534) centre (9.6901, 8.8392) ccw
  arc A2592 (77.9062, 27.7178) -> (77.9062, 27.7813) centre (77.9062, 27.7496) ccw
  line L807 (10.7296, 9.4742) -> (10.1898, 8.8392)
  arc A2593 (76.3905, 28.2892) -> (76.3905, 28.2258) centre (76.3905, 28.2575) ccw
  arc A2594 (76.708, 28.2892) -> (76.708, 28.2258) centre (76.708, 28.2575) ccw
  line L808 (10.1898, 8.8392) -> (10.8248, 8.8392)
  line L809 (77.5252, 28.2575) -> (77.9062, 28.2575)
  line L810 (9.0551, 8.8392) -> (9.0551, 9.9822)
  line L811 (9.0551, 9.9822) -> (9.3726, 9.9822)
  arc A2595 (9.3726, 9.9505) -> (9.3726, 10.014) centre (9.3726, 9.9823) ccw
  line L812 (9.6901, 8.8392) -> (9.4361, 9.3472)
  arc A2596 (9.3726, 10.014) -> (9.3726, 9.9505) centre (9.3726, 9.9823) ccw
  line L813 (77.8427, 15.1765) -> (77.8427, 14.0335)
  arc A2597 (10.1656, 8.8598) -> (10.214, 8.8186) centre (10.1898, 8.8392) ccw
  arc A2598 (76.708, 15.2083) -> (76.708, 15.1448) centre (76.708, 15.1766) ccw
  arc A2599 (76.708, 14.5733) -> (76.708, 14.5098) centre (76.708, 14.5416) ccw
  arc A2600 (10.8248, 8.8074) -> (10.8248, 8.871) centre (10.8248, 8.8392) ccw
  arc A2601 (9.3726, 9.3472) -> (9.3726, 9.9822) centre (9.3726, 9.6647) ccw
  arc A2602 (76.3588, 27.1145) -> (76.4223, 27.1145) centre (76.3906, 27.1145) ccw
  arc A2603 (10.7931, 9.6965) -> (10.8566, 9.6965) centre (10.8249, 9.6965) ccw
  arc A2604 (77.9062, 27.7495) -> (77.9062, 28.2575) centre (77.9062, 28.0035) ccw
  arc A2605 (77.9062, 27.7813) -> (77.9062, 27.7178) centre (77.9062, 27.7496) ccw
  arc A2606 (9.4645, 9.3614) -> (9.4077, 9.333) centre (9.4361, 9.3472) ccw
  arc A2607 (77.6522, 27.7813) -> (77.6522, 27.7178) centre (77.6522, 27.7496) ccw
  arc A2608 (64.633, 27.136) -> (64.5729, 27.1565) centre (64.603, 27.1462) ccw
  arc A2609 (62.611, 23.0188) -> (62.611, 23.0822) centre (62.611, 23.0505) ccw
  arc A2610 (63.9362, 23.0188) -> (63.9362, 23.0822) centre (63.9362, 23.0505) ccw
  line L814 (64.1267, 27.2415) -> (64.6347, 27.8765)
  line L815 (63.2377, 28.1305) -> (63.2377, 26.9875)
  arc A2611 (63.3965, 22.5425) -> (63.46, 22.5425) centre (63.4283, 22.5425) ccw
  arc A2612 (77.5252, 27.1462) -> (77.5252, 27.0828) centre (77.5252, 27.1145) ccw
  arc A2613 (63.46, 22.5425) -> (63.3965, 22.5425) centre (63.4283, 22.5425) ccw
  line L816 (62.9285, 21.9075) -> (62.6745, 22.4155)
  arc A2614 (63.8092, 22.5742) -> (63.8092, 22.5108) centre (63.8092, 22.5425) ccw
  arc A2615 (76.4223, 28.2575) -> (76.3588, 28.2575) centre (76.3906, 28.2575) ccw
  arc A2616 (62.611, 22.4155) -> (62.611, 23.0505) centre (62.611, 22.733) ccw
  arc A2617 (63.4282, 22.225) -> (64.0632, 22.225) centre (63.7457, 22.225) ccw
  line L817 (61.7855, 26.9875) -> (61.7855, 28.1305)
  arc A2618 (64.5729, 27.9615) -> (64.633, 27.982) centre (64.603, 27.9718) ccw
  arc A2619 (62.611, 23.0822) -> (62.611, 23.0188) centre (62.611, 23.0505) ccw
  line L818 (63.4282, 22.225) -> (63.4282, 22.5425)
  arc A2620 (64.6315, 27.9857) -> (64.5744, 27.9578) centre (64.603, 27.9717) ccw
  arc A2621 (62.7029, 22.4297) -> (62.6461, 22.4013) centre (62.6745, 22.4155) ccw
  arc A2622 (64.095, 27.559) -> (64.0315, 27.559) centre (64.0632, 27.559) ccw
  arc A2623 (62.2935, 23.0822) -> (62.2935, 23.0188) centre (62.2935, 23.0505) ccw
  arc A2624 (62.9001, 21.8933) -> (62.9569, 21.9217) centre (62.9285, 21.9075) ccw
  line L819 (64.0632, 22.2885) -> (64.0632, 22.225)
  arc A2625 (62.2935, 22.4473) -> (62.2935, 22.3838) centre (62.2935, 22.4156) ccw
  arc A2626 (63.4282, 22.5742) -> (63.4282, 22.5108) centre (63.4282, 22.5425) ccw
  line L820 (63.4282, 22.5425) -> (63.8092, 22.5425)
  arc A2627 (62.2617, 21.9075) -> (62.3253, 21.9075) centre (62.2935, 21.9075) ccw
  arc A2628 (62.3253, 23.0505) -> (62.2617, 23.0505) centre (62.2935, 23.0505) ccw
  arc A2629 (64.0632, 27.559) -> (64.1585, 27.1463) centre (65.0049, 27.5591) ccw
  arc A2630 (64.0632, 22.2885) -> (63.8092, 22.5425) centre (63.8092, 22.2885) ccw
  arc A2631 (64.5744, 27.1602) -> (64.6315, 27.1323) centre (64.603, 27.1463) ccw
  arc A2632 (64.187, 27.9578) -> (64.1299, 27.9857) centre (64.1585, 27.9717) ccw
  arc A2633 (64.603, 27.1463) -> (64.6982, 27.559) centre (63.7565, 27.5589) ccw
  arc A2634 (64.3807, 26.9875) -> (64.603, 27.1463) centre (64.3807, 27.2225) ccw
  arc A2635 (63.9362, 23.0505) -> (63.4282, 22.5425) centre (63.9362, 22.5425) ccw
  arc A2636 (64.1299, 27.1323) -> (64.187, 27.1602) centre (64.1585, 27.1462) ccw
  arc A2637 (63.3965, 22.225) -> (63.46, 22.225) centre (63.4283, 22.225) ccw
  line L821 (62.4205, 26.9875) -> (62.1665, 27.4955)
  line L822 (62.2935, 21.9075) -> (62.2935, 23.0505)
  arc A2638 (63.8092, 22.5108) -> (63.8092, 22.5742) centre (63.8092, 22.5425) ccw
  line L823 (76.3905, 28.2575) -> (76.708, 28.2575)
  arc A2639 (63.46, 22.225) -> (63.3965, 22.225) centre (63.4283, 22.225) ccw
  arc A2640 (64.095, 22.225) -> (64.0315, 22.225) centre (64.0632, 22.225) ccw
  line L824 (62.611, 22.4155) -> (62.2935, 22.4155)
  arc A2641 (62.611, 22.3838) -> (62.611, 22.4473) centre (62.611, 22.4156) ccw
  arc A2642 (77.8427, 27.7813) -> (77.8427, 27.7178) centre (77.8427, 27.7496) ccw
  arc A2643 (64.1284, 27.982) -> (64.1885, 27.9615) centre (64.1585, 27.9717) ccw
  arc A2644 (64.095, 22.2885) -> (64.0315, 22.2885) centre (64.0632, 22.2885) ccw
  arc A2645 (62.9004, 27.9013) -> (62.94, 27.8517) centre (62.9202, 27.8765) ccw
  arc A2646 (61.7855, 27.5272) -> (61.7855, 27.4638) centre (61.7855, 27.4955) ccw
  arc A2647 (63.5552, 26.9558) -> (63.5552, 27.0192) centre (63.5552, 26.9875) ccw
  arc A2648 (76.708, 27.6225) -> (76.708, 28.2575) centre (76.708, 27.94) ccw
  arc A2649 (62.611, 22.4473) -> (62.611, 22.3838) centre (62.611, 22.4156) ccw
  line L825 (77.0255, 27.1145) -> (76.7715, 27.6225)
  arc A2650 (64.0315, 22.2885) -> (64.095, 22.2885) centre (64.0632, 22.2885) ccw
  arc A2651 (64.3807, 26.9558) -> (64.3807, 27.0192) centre (64.3807, 26.9875) ccw
  line L826 (61.7855, 28.1305) -> (62.103, 28.1305)
  arc A2652 (62.103, 28.0988) -> (62.103, 28.1623) centre (62.103, 28.1305) ccw
  arc A2653 (61.7538, 26.9875) -> (61.8173, 26.9875) centre (61.7856, 26.9875) ccw
  arc A2654 (76.3905, 27.6543) -> (76.3905, 27.5908) centre (76.3905, 27.6226) ccw
  arc A2655 (64.0315, 22.225) -> (64.095, 22.225) centre (64.0632, 22.225) ccw
  line L827 (62.2935, 23.0505) -> (62.611, 23.0505)
  arc A2656 (62.1949, 27.5097) -> (62.1381, 27.4813) centre (62.1665, 27.4955) ccw
  arc A2657 (44.577, 36.0998) -> (44.577, 36.1633) centre (44.577, 36.1316) ccw
  arc A2658 (64.0315, 27.559) -> (64.095, 27.559) centre (64.0632, 27.559) ccw
  line L828 (44.8945, 35.6235) -> (44.6405, 36.1315)
  arc A2659 (44.577, 36.7347) -> (44.577, 36.7983) centre (44.577, 36.7665) ccw
  arc A2660 (45.7315, 36.7417) -> (45.6919, 36.7913) centre (45.7117, 36.7665) ccw
  arc A2661 (44.2595, 36.7983) -> (44.2595, 36.7347) centre (44.2595, 36.7665) ccw
  line L829 (62.9202, 27.8765) -> (63.2377, 28.1305)
  line L830 (62.9202, 26.9875) -> (63.5552, 26.9875)
  arc A2662 (61.7855, 28.1623) -> (61.7855, 28.0988) centre (61.7855, 28.1305) ccw
  line L831 (44.2595, 35.6235) -> (44.2595, 36.7665)
  line L832 (44.577, 36.1315) -> (44.2595, 36.1315)
  line L833 (46.5372, 35.6235) -> (46.8547, 35.6235)
  arc A2663 (44.2595, 36.1633) -> (44.2595, 36.0998) centre (44.2595, 36.1316) ccw
  arc A2664 (64.1585, 27.1463) -> (64.3807, 26.9875) centre (64.3807, 27.2224) ccw
  arc A2665 (64.6595, 27.8567) -> (64.6099, 27.8963) centre (64.6347, 27.8765) ccw
  arc A2666 (64.3807, 28.1305) -> (64.1585, 27.9718) centre (64.3807, 27.8956) ccw
  arc A2667 (44.6322, 30.3848) -> (44.6322, 30.4483) centre (44.6322, 30.4166) ccw
  arc A2668 (45.3744, 36.5373) -> (45.414, 36.4877) centre (45.3942, 36.5125) ccw
  arc A2669 (46.5372, 35.6553) -> (46.5372, 35.5917) centre (46.5372, 35.6235) ccw
  arc A2670 (44.6689, 36.1457) -> (44.6121, 36.1173) centre (44.6405, 36.1315) ccw
  arc A2671 (45.68, 35.6235) -> (45.7435, 35.6235) centre (45.7118, 35.6235) ccw
  arc A2672 (44.2278, 35.6235) -> (44.2913, 35.6235) centre (44.2596, 35.6235) ccw
  arc A2673 (62.103, 27.5272) -> (62.103, 27.4638) centre (62.103, 27.4955) ccw
  arc A2674 (64.3807, 28.0988) -> (64.3807, 28.1623) centre (64.3807, 28.1305) ccw
  line L834 (44.3147, 31.5595) -> (44.3147, 30.4165)
  arc A2675 (64.3807, 28.1623) -> (64.3807, 28.0988) centre (64.3807, 28.1305) ccw
  arc A2676 (64.3807, 27.0192) -> (64.3807, 26.9558) centre (64.3807, 26.9875) ccw
  arc A2677 (62.3921, 26.9733) -> (62.4489, 27.0017) centre (62.4205, 26.9875) ccw
  arc A2678 (64.73, 27.559) -> (64.6665, 27.559) centre (64.6983, 27.559) ccw
  arc A2679 (46.0292, 35.5917) -> (46.0292, 35.6553) centre (46.0292, 35.6235) ccw
  arc A2680 (46.8547, 35.6235) -> (46.8547, 36.2585) centre (46.8547, 35.941) ccw
  arc A2681 (62.9202, 27.0192) -> (62.9202, 26.9558) centre (62.9202, 26.9875) ccw
  arc A2682 (63.206, 26.9875) -> (63.2695, 26.9875) centre (63.2378, 26.9875) ccw
  arc A2683 (64.603, 27.9718) -> (64.3807, 28.1305) centre (64.3808, 27.8956) ccw
  arc A2684 (61.8173, 28.1305) -> (61.7538, 28.1305) centre (61.7856, 28.1305) ccw
  arc A2685 (44.8661, 35.6093) -> (44.9229, 35.6377) centre (44.8945, 35.6235) ccw
  arc A2686 (63.2575, 28.1057) -> (63.2179, 28.1553) centre (63.2377, 28.1305) ccw
  line L835 (45.3942, 36.5125) -> (45.7117, 36.7665)
  arc A2687 (63.2695, 28.1305) -> (63.206, 28.1305) centre (63.2378, 28.1305) ccw
  arc A2688 (62.103, 28.1623) -> (62.103, 28.0988) centre (62.103, 28.1305) ccw
  line L836 (45.7117, 36.7665) -> (45.7117, 35.6235)
  arc A2689 (64.1585, 27.9718) -> (64.0632, 27.559) centre (65.0052, 27.5589) ccw
  arc A2690 (45.3942, 35.6553) -> (45.3942, 35.5917) centre (45.3942, 35.6235) ccw
  arc A2691 (45.7435, 36.7665) -> (45.68, 36.7665) centre (45.7118, 36.7665) ccw
  arc A2692 (64.1019, 27.2613) -> (64.1515, 27.2217) centre (64.1267, 27.2415) ccw
  arc A2693 (62.103, 27.4638) -> (62.103, 27.5272) centre (62.103, 27.4955) ccw
  arc A2694 (64.1885, 27.1565) -> (64.1284, 27.136) centre (64.1585, 27.1462) ccw
  arc A2695 (43.9972, 30.4483) -> (43.9972, 30.3848) centre (43.9972, 30.4166) ccw
  arc A2696 (44.577, 36.1633) -> (44.577, 36.0998) centre (44.577, 36.1316) ccw
  line L837 (44.2595, 36.7665) -> (44.577, 36.7665)
  arc A2697 (44.577, 36.7983) -> (44.577, 36.7347) centre (44.577, 36.7665) ccw
  arc A2698 (44.2913, 36.7665) -> (44.2278, 36.7665) centre (44.2596, 36.7665) ccw
  arc A2699 (62.103, 27.4955) -> (62.103, 28.1305) centre (62.103, 27.813) ccw
  line L838 (45.3942, 35.6235) -> (46.0292, 35.6235)
  arc A2700 (46.8547, 35.5917) -> (46.8547, 35.6553) centre (46.8547, 35.6235) ccw
  arc A2701 (64.6665, 27.559) -> (64.73, 27.559) centre (64.6983, 27.559) ccw
  line L839 (62.103, 27.4955) -> (61.7855, 27.4955)
  arc A2702 (44.577, 36.1315) -> (44.577, 36.7665) centre (44.577, 36.449) ccw
  arc A2703 (64.6982, 27.559) -> (64.603, 27.9718) centre (63.7563, 27.5592) ccw
  arc A2704 (46.9182, 36.7983) -> (46.9182, 36.7347) centre (46.9182, 36.7665) ccw
  arc A2705 (44.323, 44.6088) -> (44.323, 44.6723) centre (44.323, 44.6406) ccw
  arc A2706 (44.0055, 44.6723) -> (44.0055, 44.6088) centre (44.0055, 44.6406) ccw
  arc A2707 (45.1402, 43.5293) -> (45.1402, 43.4657) centre (45.1402, 43.4975) ccw
  arc A2708 (46.9182, 43.7197) -> (46.9182, 43.7833) centre (46.9182, 43.7515) ccw
  arc A2709 (46.696, 43.4975) -> (46.7595, 43.4975) centre (46.7278, 43.4975) ccw
  arc A2710 (46.9182, 36.2585) -> (46.9182, 36.7665) centre (46.9182, 36.5125) ccw
  line L840 (31.1702, 44.3865) -> (31.4877, 44.6405)
  arc A2711 (30.4449, 44.0197) -> (30.3881, 43.9913) centre (30.4165, 44.0055) ccw
  arc A2712 (30.6421, 43.4833) -> (30.6989, 43.5117) centre (30.6705, 43.4975) ccw
  arc A2713 (31.5075, 44.6157) -> (31.4679, 44.6653) centre (31.4877, 44.6405) ccw
  arc A2714 (45.4775, 44.6157) -> (45.4379, 44.6653) centre (45.4577, 44.6405) ccw
  line L841 (45.4577, 44.6405) -> (45.4577, 43.4975)
  line L842 (44.323, 44.0055) -> (44.0055, 44.0055)
  arc A2715 (44.0055, 44.0373) -> (44.0055, 43.9738) centre (44.0055, 44.0055) ccw
  arc A2716 (44.4149, 44.0197) -> (44.3581, 43.9913) centre (44.3865, 44.0055) ccw
  arc A2717 (43.9738, 43.4975) -> (44.0373, 43.4975) centre (44.0055, 43.4975) ccw
  arc A2718 (44.323, 44.0373) -> (44.323, 43.9738) centre (44.323, 44.0055) ccw
  arc A2719 (46.9182, 36.7347) -> (46.9182, 36.7983) centre (46.9182, 36.7665) ccw
  arc A2720 (46.8547, 35.6553) -> (46.8547, 35.5917) centre (46.8547, 35.6235) ccw
  arc A2721 (46.9182, 36.2268) -> (46.9182, 36.2903) centre (46.9182, 36.2585) ccw
  arc A2722 (44.6121, 43.4833) -> (44.6689, 43.5117) centre (44.6405, 43.4975) ccw
  arc A2723 (44.323, 43.9738) -> (44.323, 44.0373) centre (44.323, 44.0055) ccw
  arc A2724 (45.4895, 44.6405) -> (45.426, 44.6405) centre (45.4577, 44.6405) ccw
  arc A2725 (46.2832, 43.7833) -> (46.2832, 43.7197) centre (46.2832, 43.7515) ccw
  line L843 (44.6405, 43.4975) -> (44.3865, 44.0055)
  arc A2726 (46.9182, 36.2903) -> (46.9182, 36.2268) centre (46.9182, 36.2585) ccw
  line L844 (46.5372, 44.6405) -> (46.2832, 43.7515)
  arc A2727 (30.0355, 44.0373) -> (30.0355, 43.9738) centre (30.0355, 44.0055) ccw
  arc A2728 (30.0355, 44.6723) -> (30.0355, 44.6088) centre (30.0355, 44.6406) ccw
  line L845 (44.0055, 44.6405) -> (44.323, 44.6405)
  line L846 (45.1402, 44.3865) -> (45.4577, 44.6405)
  arc A2729 (46.8547, 36.2903) -> (46.8547, 36.2268) centre (46.8547, 36.2585) ccw
  arc A2730 (46.5372, 36.7983) -> (46.5372, 36.7347) centre (46.5372, 36.7665) ccw
  arc A2731 (46.5677, 44.6318) -> (46.5067, 44.6492) centre (46.5372, 44.6405) ccw
  line L847 (46.2832, 43.7515) -> (46.9182, 43.7515)
  line L848 (46.9182, 36.2585) -> (46.6642, 36.2585)
  arc A2732 (31.1504, 44.4113) -> (31.19, 44.3617) centre (31.1702, 44.3865) ccw
  arc A2733 (46.2527, 43.7602) -> (46.3137, 43.7428) centre (46.2832, 43.7515) ccw
  line L849 (31.4877, 44.6405) -> (31.4877, 43.4975)
  arc A2734 (45.7752, 43.4657) -> (45.7752, 43.5293) centre (45.7752, 43.4975) ccw
  arc A2735 (44.323, 44.6723) -> (44.323, 44.6088) centre (44.323, 44.6406) ccw
  arc A2736 (31.5195, 44.6405) -> (31.456, 44.6405) centre (31.4878, 44.6405) ccw
  line L850 (46.7277, 44.0055) -> (46.7277, 43.4975)
  line L851 (31.1702, 43.4975) -> (31.8052, 43.4975)
  line L852 (46.5372, 36.7665) -> (46.9182, 36.7665)
  arc A2737 (44.0373, 44.6405) -> (43.9738, 44.6405) centre (44.0055, 44.6405) ccw
  arc A2738 (46.7595, 44.0055) -> (46.696, 44.0055) centre (46.7278, 44.0055) ccw
  arc A2739 (45.1204, 44.4113) -> (45.16, 44.3617) centre (45.1402, 44.3865) ccw
  arc A2740 (30.353, 44.6723) -> (30.353, 44.6088) centre (30.353, 44.6406) ccw
  line L853 (30.6705, 43.4975) -> (30.4165, 44.0055)
  arc A2741 (45.426, 43.4975) -> (45.4895, 43.4975) centre (45.4577, 43.4975) ccw
  arc A2742 (30.0673, 44.6405) -> (30.0038, 44.6405) centre (30.0356, 44.6405) ccw
  line L854 (45.1402, 43.4975) -> (45.7752, 43.4975)
  arc A2743 (46.6642, 36.2903) -> (46.6642, 36.2268) centre (46.6642, 36.2585) ccw
  line L855 (44.0055, 43.4975) -> (44.0055, 44.6405)
  arc A2744 (30.353, 43.9738) -> (30.353, 44.0373) centre (30.353, 44.0055) ccw
  arc A2745 (30.0038, 43.4975) -> (30.0673, 43.4975) centre (30.0356, 43.4975) ccw
  arc A2746 (31.456, 43.4975) -> (31.5195, 43.4975) centre (31.4878, 43.4975) ccw
  line L856 (30.353, 44.0055) -> (30.0355, 44.0055)
  arc A2747 (44.323, 44.0055) -> (44.323, 44.6405) centre (44.323, 44.323) ccw
  line L857 (30.0355, 44.6405) -> (30.353, 44.6405)
  arc A2748 (8.763, 17.1768) -> (8.763, 17.2402) centre (8.763, 17.2085) ccw
  arc A2749 (8.8549, 17.2227) -> (8.7981, 17.1943) centre (8.8265, 17.2085) ccw
  arc A2750 (11.39, 17.018) -> (11.3265, 17.018) centre (11.3582, 17.018) ccw
  arc A2751 (9.5604, 17.6143) -> (9.6, 17.5647) centre (9.5802, 17.5895) ccw
  arc A2752 (10.6915, 17.3355) -> (10.755, 17.3355) centre (10.7233, 17.3355) ccw
  line L858 (32.3132, 44.1325) -> (32.3132, 44.6405)
  arc A2753 (32.6942, 43.4975) -> (32.9482, 43.7515) centre (32.6942, 43.7515) ccw
  arc A2754 (32.9165, 43.7515) -> (32.98, 43.7515) centre (32.9483, 43.7515) ccw
  arc A2755 (8.763, 17.2085) -> (8.763, 17.8435) centre (8.763, 17.526) ccw
  arc A2756 (32.98, 43.7515) -> (32.9165, 43.7515) centre (32.9483, 43.7515) ccw
  line L859 (32.3132, 43.4975) -> (32.6942, 43.4975)
  arc A2757 (82.3874, 4.699) -> (82.6414, 4.953) centre (82.3874, 4.953) ccw
  arc A2758 (30.353, 44.0373) -> (30.353, 43.9738) centre (30.353, 44.0055) ccw
  arc A2759 (32.6942, 43.5293) -> (32.6942, 43.4657) centre (32.6942, 43.4975) ccw
  arc A2760 (32.345, 44.6405) -> (32.2815, 44.6405) centre (32.3133, 44.6405) ccw
  line L860 (9.0805, 16.7005) -> (8.8265, 17.2085)
  line L861 (11.3582, 17.0815) -> (11.3582, 17.018)
  arc A2761 (31.1702, 43.5293) -> (31.1702, 43.4657) centre (31.1702, 43.4975) ccw